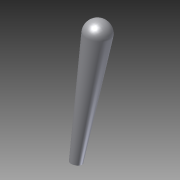
# Autodesk Inventor part: WT_toggle
Saved by Autodesk Inventor 2011 SP1 (Build 150282100, 282)
## iProperties
Created: 2013-12-24
Part Number: WT_toggle
Catalog Web Link: www.cadenas.de
Description: WT Toggle-WT Toggle
Vendor: NKKSWITCHES
Document SubType Name: Modeling
Designer: PARTuser1
Manufacturer: NKKSWITCHES
Density: 1 g/cm^3
Category: PARTsolutions
Company: NKKSWITCHES
Title: WT_toggle
Author: Cadenas PARTsolutions
Comments: WT Toggle
PSOL_IDENT_0: {$CADENAS_DATA\23d-libs\nkkswitches\toggle\wt\parts\wt_toggle.prj},163 {VTYP=3D},{NB=WT_toggle},{LIN
PSOL_IDENT_1: A=WT_toggle},{NN=WT Toggle},{DATE=24.06.2008 05:17:41},{GEOMDATE=23.06.2008 11:37:00},{VERSION=},{LI
PSOL_IDENT_2: NEID=10},{LINESUBID=-1},{WBVAR=}  {NB=WT_toggle},{LINA=WT_toggle},{KT=DUMMY},{PN=WT_toggle},{D=0.224
PSOL_IDENT_3: 0}
CNS_NN: WT Toggle
CNS_NT: WT Toggle
CNS_NB: WT_toggle
CNS_NBSYN: $PN.
CNS_LINA: WT_toggle
CNS_PN: WT_toggle
CNS_D: 0.2240
SUPPLIER: NKKSWITCHES
ARTICLENO: WT_toggle
BOMINFO: WT_toggle
CREATOR: CADENAS GmbH
Autodesk Inventor part; units mm, degrees
sketch "Sketch_1" plane through (0, 0, 0) normal (1, 0, 0) x (0, 1, 0)
  line L0 (-1.1898, 0.7631) -> (26.562, -5.1357)
  arc A0 (23.0171, -7.285) -> (26.562, -5.1357) centre (23.7794, -4.5443) ccw
  line L1 (23.0171, -7.285) -> (-1.4538, -0.4791)
  line L2 (-1.4538, -0.4791) -> (-1.1898, 0.7631)
  line L3 (-1.1898, 0.7631) -> (26.562, -5.1357)
  constraints: 8 end point, 2 point on circle, 1 centre point
revolve "Revolution1" add sketch "Sketch_1" angle 360 about axis through (0, -1.1898, 0.7631) along (0, 0.9781476, -0.2079117)
ref_plane "toggle_XY" through (0, 2.4003, 0) normal (0, 1, 0) x (1, 0, 0)
ref_plane "toggle_YZ" through (0, 2.4003, 0) normal (1, 0, 0) x (0, 0, -1)
ref_plane "toggle_ZX" through (0, 2.4003, 0) normal (0, 0, -1) x (0, 1, 0)
body "Solid1"
